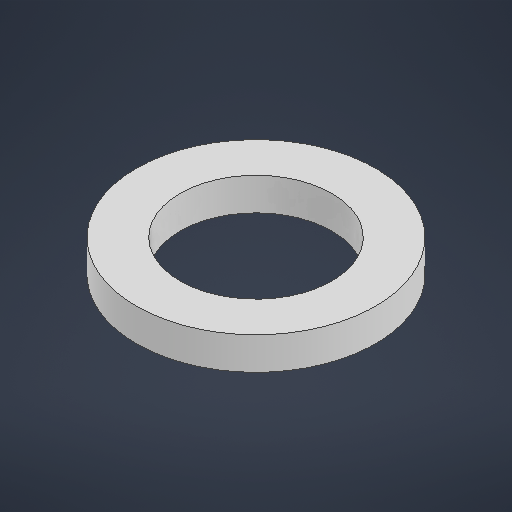
# Autodesk Inventor part: exterior_rodamiento
Saved by Autodesk Inventor 2026.2 (Build 302298010, 298A)
## iProperties
Created: 2026-06-02
Part Number: exterior_rodamiento
Material: Genérico
Document SubType Name: Modeling
Designer: agusb
Density: 1 g/cm^3
Appearance: Valor por defecto
Author: agusb
Autodesk Inventor part; units mm, degrees
ref_plane "YZ Plane" through (0, 0, 0) normal (1, 0, 0) x (0, 1, 0)
ref_plane "XZ Plane" through (0, 0, 0) normal (0, 1, 0) x (-1, 0, 0)
ref_plane "XY Plane" through (0, 0, 0) normal (0, 0, 1) x (1, 0, 0)
sketch "Boceto1" plane through (0, 0, 0) normal (0, 1, 0) x (-1, 0, 0)
  circle A0 centre (0, 0) radius 82.5
  circle A1 centre (0, 0) radius 130
  dimension "d0" = 165
  dimension "d1" = 260
  constraints: 2 centre point, 2 coincident
  measures "d0" diameter of A0
  measures "d1" diameter of A1
extrude "Extrusión1" add sketch "Boceto1" along normal blind 35.4
